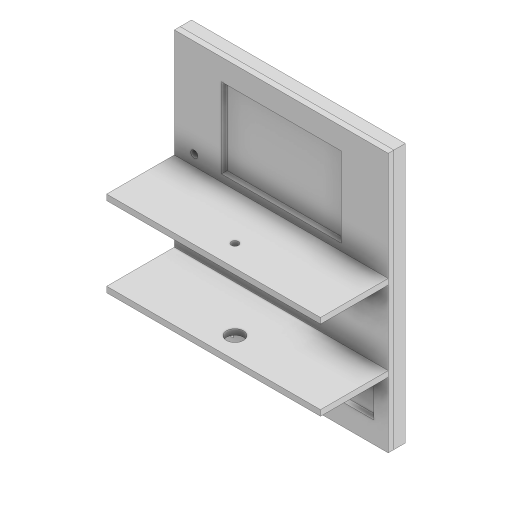
# Autodesk Inventor part: Деталь2
Saved by Autodesk Inventor 2023 (Build 270158000, 158)
## iProperties
Created: 2022-09-27
Part Number: Деталь2
Material: Типовые
Document SubType Name: Modeling
Designer: Admin
Density: 1 g/cm^3
Appearance: По умолчанию
Author: Admin
Autodesk Inventor part; units mm, degrees
ref_plane "YZ Plane" through (0, 0, 0) normal (1, 0, 0) x (0, 1, 0)
sketch "Эскиз1" plane through (0, 0, 0) normal (0, 0, 1) x (1, 0, 0)
  line L0 (-75, 91) -> (75, 91)
  line L1 (75, 91) -> (75, -91)
  line L2 (75, -91) -> (-75, -91)
  line L3 (-75, -91) -> (-75, 91)
  line L4 (-75, 91) -> (75, -91) construction
  line L5 (75, 91) -> (-75, -91) construction
  line L6 (-25, -55) -> (65, -55)
  line L7 (65, -55) -> (65, -76)
  line L8 (65, -76) -> (-25, -76)
  line L9 (-25, -76) -> (-25, -55)
  line L10 (-57, -73) -> (-65, -73)
  line L11 (-65, -73) -> (-65, -58)
  line L12 (-65, -58) -> (-57, -58)
  line L13 (-57, -58) -> (-57, -73)
  line L14 (-75, -41) -> (75, -41)
  line L15 (-75, 11) -> (75, 11)
  line L16 (-42, 76) -> (42, 76)
  line L17 (42, 76) -> (42, 20)
  line L18 (42, 20) -> (-42, 20)
  line L19 (-42, 20) -> (-42, 76)
  line L20 (-75, 15) -> (75, 15)
  line L21 (-75, -45) -> (75, -45)
  line L22 (-55, 15) -> (-55, 11)
  line L23 (-35, 15) -> (-35, 11)
  line L24 (-10, 15) -> (-10, 11)
  line L25 (10, 15) -> (10, 11)
  line L26 (35, 15) -> (35, 11)
  line L27 (55, 15) -> (55, 11)
  line L28 (0, 15) -> (0, 11) construction
  line L29 (-75, -15) -> (75, -15) construction
  line L30 (-55, -45) -> (-55, -41)
  line L31 (-35, -45) -> (-35, -41)
  line L32 (-10, -45) -> (-10, -41)
  line L33 (10, -45) -> (10, -41)
  line L34 (35, -45) -> (35, -41)
  line L35 (55, -45) -> (55, -41)
  line L36 (-33.75, -55.5) -> (-48.25, -55.5)
  line L37 (-48.25, -55.5) -> (-48.25, -75.5)
  line L38 (-48.25, -75.5) -> (-33.75, -75.5)
  line L39 (-33.75, -75.5) -> (-33.75, -55.5)
  line L40 (-41, -75.5) -> (-41, -55.5) construction
  circle A0 centre (-61, 22.5) radius 2.5
  circle A1 centre (-61, -51.5) radius 2.5
  point P0 (0, 0)
  point P1 (-57, -65.5)
  point P2 (-25, -65.5)
  point P3 (0, 76)
  point P4 (0, 91)
  point P5 (55, -41)
  point P6 (55, -45)
  point P7 (35, -45)
  point P8 (35, -41)
  point P9 (-10, -41)
  point P10 (10, -41)
  point P11 (10, -45)
  point P12 (-10, -45)
  point P13 (-55, -41)
  point P14 (-35, -41)
  point P15 (-35, -45)
  point P16 (-55, -45)
  point P17 (-33.75, -65.5)
  point P18 (-61, -58)
  dimension "d15" = 4
  dimension "d1" = 150
  dimension "d2" = 90
  dimension "d3" = 21
  dimension "d4" = 8
  dimension "d5" = 15
  dimension "d6" = 52
  dimension "d7" = 56
  dimension "d8" = 84
  dimension "d9" = 15
  dimension "d10" = 10
  dimension "d11" = 10
  dimension "d12" = 15
  dimension "d13" = 14
  dimension "d14" = 9
  dimension "d16" = 4
  dimension "d19" = 20
  dimension "d20" = 20
  dimension "d21" = 20
  dimension "d38" = 20
  dimension "d39" = 14.5
  dimension "d47" = 5
  dimension "d48" = 5
  dimension "d49" = 7.5
  dimension "d50" = 14
  dimension "d51" = 14
  dimension "d52" = 6.5
  constraints: 78 end point, 12 symmetric about line, 11 parallel, 10 midpoint, 10 point on line, 8 perpendicular, 8 vertical, 5 horizontal, 2 centre point, 2 horizontal alignment, 1 vertical alignment, 24 other
  measures "d1" distance of L1.end L2.end
  measures "d2" distance of L6.start L6.end
  measures "d3" distance of L6.end L7.end
  measures "d4" distance of L11.end L12.end
  measures "d5" distance of L12.end L10.start
  measures "d7" distance between parallel lines of L16 L18
  measures "d8" distance of L16.start L16.end
  measures "d9" distance between parallel lines of L8 L2
  measures "d10" distance between parallel lines of L1 L7
  measures "d11" distance between parallel lines of L3 L11
  measures "d12" distance between parallel lines of L0 L16
  measures "d13" distance between parallel lines of L14 L6
  measures "d16" distance between parallel lines of L14 L21
  measures "d19" distance between parallel lines of L23 L22
  measures "d20" distance between parallel lines of L3 L22
  measures "d21" distance between parallel lines of L25 L24
  measures "d38" distance of L38.end L36.start
  measures "d39" distance of L37.end L38.end
  measures "d47" diameter of A1
  measures "d48" diameter of A0
  measures "d50" distance from line of L3 A0.centre
  measures "d51" distance from line of L3 A1.centre
  measures "d52" distance from line of L21 A1.centre
extrude "Выдавливание1" add sketch "Эскиз1" against normal blind 4 contours L0 L1 L20 L3 | L20 L22 L15 L3 | L1 L15 L27 L20 | L15 L1 L14 L3 | L14 L30 L21 L3 | L20 L24 L15 L23 | L1 L21 L35 L14 | L26 L15 L25 L20 | L21 L1 L2 L3 | L14 L32 L21 L31 | L34 L21 L33 L14
sketch "Эскиз2" plane through (-10, 11, 0) normal (0, 1, 0) x (1, 0, 0)
  line L0 (-65, 0) -> (85, 0) projected
  line L1 (85, 0) -> (-65, 0)
  line L2 (-65, 0) -> (-65, -47.5)
  line L3 (-65, -47.5) -> (85, -47.5)
  line L4 (85, -47.5) -> (85, 0)
  circle A0 centre (10, -32.5) radius 2.5
  line L5 (8.8126, -34.7) -> (11.1874, -34.7)
  line L6 (8.8126, -30.3) -> (11.1874, -30.3)
  line L7 (7.5, -32.5) -> (12.5, -32.5) construction
  point P0 (10, 0)
  point P1 (10, -47.5)
  dimension "d22" = 5
  dimension "d23" = 32.5
  dimension "d24" = 15
  dimension "d44" = 4.4
  constraints: 14 end point, 6 point on circle, 4 parallel, 2 horizontal, 2 midpoint, 1 centre point, 1 perpendicular, 1 vertical alignment, 1 other
  measures "d22" diameter of A0
  measures "d23" distance from line of L0 A0.centre
  measures "d24" distance from line of L3 A0.centre
  measures "d44" distance between parallel lines of L5 L6
extrude "Выдавливание2" add sketch "Эскиз2" along normal blind 4 separate body contours L0 L4 L3 L2 | L6 A0 | A0 L5
extrude "Выдавливание4" add sketch "Эскиз1" against normal blind 4 contours L20 L23 L15 L22 | L27 L15 L26 L20 | L20 L25 L15 L24 bodies 2
ref_plane "РабПлоскость1" through (-75, -15, 0) normal (0, -1, 0) x (1, 0, 0)
mirror "Зеркальное отражение2" about plane through (-75, -15, 0) normal (0, -1, 0) of "Выдавливание2", "Выдавливание4" bodies 2
sketch "Эскиз9" plane through (-75, -41, 47.5) normal (0, 1, 0) x (1, 0, 0)
  arc A0 (76.1874, 12.8) -> (76.1874, 17.2) centre (75, 15) ccw projected
  circle A1 centre (75, 15) radius 6
  point P0 (75, 47.5)
  dimension "d35" = 12
  constraints: 1 centre point, 1 coincident
  measures "d35" diameter of A1
extrude "Выдавливание6" cut sketch "Эскиз9" against normal through all bodies 2
sketch "Основание" plane through (0, 0, -4) normal (0, 0, -1) x (-1, 0, 0)
  line L0 (75, 91) -> (-75, 91) projected
  line L1 (-75, 91) -> (-75, -91) projected
  line L2 (-75, -91) -> (75, -91) projected
  line L3 (75, -91) -> (75, 91) projected
  line L4 (-55, -45) -> (-55, -41) projected
  line L5 (-55, -41) -> (-35, -41) projected
  line L6 (-35, -41) -> (-35, -45) projected
  line L7 (-35, -45) -> (-55, -45) projected
  line L8 (-35, 11) -> (-55, 11) projected
  line L9 (-55, 11) -> (-55, 15) projected
  line L10 (-55, 15) -> (-35, 15) projected
  line L11 (-35, 15) -> (-35, 11) projected
  line L12 (55, 15) -> (55, 11) projected
  line L13 (55, 11) -> (35, 11) projected
  line L14 (35, 11) -> (35, 15) projected
  line L15 (35, 15) -> (55, 15) projected
  line L16 (-42, 76) -> (42, 76) projected
  line L17 (42, 76) -> (42, 20) projected
  line L18 (42, 20) -> (-42, 20) projected
  line L19 (-42, 20) -> (-42, 76) projected
  line L20 (10, 15) -> (10, 11) projected
  line L21 (10, 11) -> (-10, 11) projected
  line L22 (-10, 11) -> (-10, 15) projected
  line L23 (-10, 15) -> (10, 15) projected
  line L24 (35, -41) -> (55, -41) projected
  line L25 (55, -41) -> (55, -45) projected
  line L26 (55, -45) -> (35, -45) projected
  line L27 (35, -45) -> (35, -41) projected
  line L28 (-10, -41) -> (10, -41) projected
  line L29 (10, -41) -> (10, -45) projected
  line L30 (10, -45) -> (-10, -45) projected
  line L31 (-10, -45) -> (-10, -41) projected
  line L32 (33.75, -75.5) -> (33.75, -55.5) projected
  line L33 (33.75, -55.5) -> (48.25, -55.5) projected
  line L34 (48.25, -55.5) -> (48.25, -75.5) projected
  line L35 (48.25, -75.5) -> (33.75, -75.5) projected
  line L36 (65, -73) -> (57, -73) projected
  line L37 (57, -73) -> (57, -58) projected
  line L38 (57, -58) -> (65, -58) projected
  line L39 (65, -58) -> (65, -73) projected
  line L40 (-65, -55) -> (25, -55) projected
  line L41 (25, -55) -> (25, -76) projected
  line L42 (25, -76) -> (-65, -76) projected
  line L43 (-65, -76) -> (-65, -55) projected
  point P0 (0, 0)
sketch "Стенка с фоторезистором" plane through (-10, 15, 0) normal (0, 1, 0) x (1, 0, 0)
  line L0 (85, 0) -> (65, 0) projected
  line L1 (65, 0) -> (65, 4) projected
  line L2 (45, 4) -> (65, 4) projected
  line L3 (45, 0) -> (45, 4) projected
  line L4 (45, 0) -> (20, 0) projected
  line L5 (20, 0) -> (20, 4) projected
  line L6 (0, 4) -> (20, 4) projected
  line L7 (0, 0) -> (0, 4) projected
  line L8 (0, 0) -> (-25, 0) projected
  line L9 (-25, 0) -> (-25, 4) projected
  line L10 (-45, 4) -> (-25, 4) projected
  line L11 (-45, 0) -> (-45, 4) projected
  line L12 (-45, 0) -> (-65, 0) projected
  line L13 (-65, 0) -> (-65, -47.5) projected
  line L14 (-65, -47.5) -> (85, -47.5) projected
  line L15 (85, -47.5) -> (85, 0) projected
  arc A0 (11.1874, -34.7) -> (11.1874, -30.3) centre (10, -32.5) ccw projected
  line L16 (11.1874, -34.7) -> (8.8126, -34.7) projected
  arc A1 (8.8126, -30.3) -> (8.8126, -34.7) centre (10, -32.5) ccw projected
  line L17 (8.8126, -30.3) -> (11.1874, -30.3) projected
  point P0 (10, 0)
sketch "Стенка с лазером" plane through (-75, -45, 47.5) normal (0, -1, 0) x (1, 0, 0)
  circle A0 centre (75, -15) radius 6 projected
  line L0 (150, -47.5) -> (130, -47.5) projected
  line L1 (150, 0) -> (150, -47.5) projected
  line L2 (0, 0) -> (150, 0) projected
  line L3 (0, -47.5) -> (0, 0) projected
  line L4 (20, -47.5) -> (0, -47.5) projected
  line L5 (20, -47.5) -> (20, -51.5) projected
  line L6 (20, -51.5) -> (40, -51.5) projected
  line L7 (40, -47.5) -> (40, -51.5) projected
  line L8 (65, -47.5) -> (40, -47.5) projected
  line L9 (65, -47.5) -> (65, -51.5) projected
  line L10 (65, -51.5) -> (85, -51.5) projected
  line L11 (85, -47.5) -> (85, -51.5) projected
  line L12 (110, -47.5) -> (85, -47.5) projected
  line L13 (110, -47.5) -> (110, -51.5) projected
  line L14 (110, -51.5) -> (130, -51.5) projected
  line L15 (130, -47.5) -> (130, -51.5) projected
  point P0 (75, -47.5)
sketch "Поддон" plane through (0, 0, -4) normal (0, 0, -1) x (-1, 0, 0)
  line L0 (-75, -91) -> (75, -91) projected
  line L1 (75, -91) -> (75, 91) projected
  line L2 (75, 91) -> (-75, 91) projected
  line L3 (-75, 91) -> (-75, -91) projected
  circle A0 centre (61, 22.5) radius 2.5 projected
  circle A1 centre (61, -51.5) radius 2.5 projected
  line L4 (63.5, 22.5) -> (63.5, -51.5)
  circle A2 centre (61, 22.5) radius 2.5 projected
  line L5 (58.5, 22.5) -> (58.5, -51.5)
  point P0 (0, 0)
  constraints: 4 end point, 4 tangent, 3 point on circle
sketch "Эскиз16" plane through (-10, 11, 0) normal (0, -1, 0) x (1, 0, 0)
  arc A0 (8.8126, 34.7) -> (8.8126, 30.3) centre (10, 32.5) ccw projected
  circle A1 centre (10, 32.5) radius 2.5
  point P0 (10, 0)
  point P1 (8.8126, 30.3)
  point P2 (8.8126, 34.7)
  constraints: 1 centre point, 1 coincident, 1 concentric
extrude "Выдавливание7" cut sketch "Эскиз16" against normal through all bodies 2
extrude "Выдавливание8" add sketch "Поддон" along normal blind 8 separate body
sketch "Эскиз17" plane through (0, 0, -12) normal (0, 0, -1) x (-1, 0, 0)
  line L0 (75, -91) -> (75, 91) projected
  line L1 (75, 91) -> (-75, 91) projected
  line L2 (-75, 91) -> (-75, -91) projected
  line L3 (-75, -91) -> (75, -91) projected
  line L4 (63.5, 22.5) -> (63.5, -51.5) projected
  arc A0 (58.5, -51.5) -> (63.5, -51.5) centre (61, -51.5) ccw projected
  line L5 (58.5, -51.5) -> (58.5, 22.5) projected
  arc A1 (63.5, 22.5) -> (58.5, 22.5) centre (61, 22.5) ccw projected
  point P0 (0, 0)
extrude "Выдавливание9" add sketch "Эскиз17" against normal blind 4 contours L4 A0 L5 A1 bodies 3
ref_plane "РабПлоскость2" through (-10, -4.5, 0) normal (0, -1, 0) x (1, 0, 0)
split body "Разделение1" result two bodies by plane through (-10, -4.5, 0) normal (0, -1, 0) bodies 2 first body at (-38.6667, -41.5, 26.6667)
